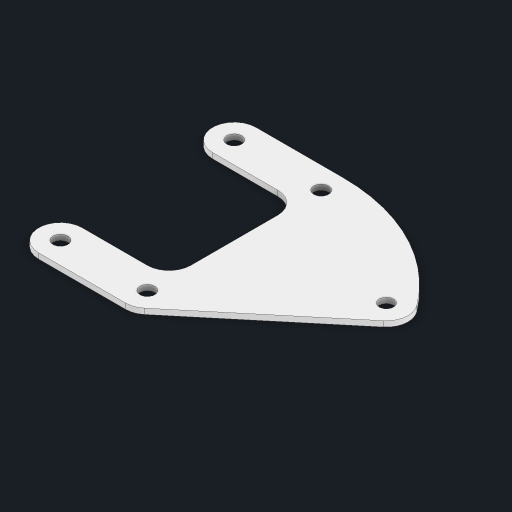
# Autodesk Inventor part: gusset
Saved by Autodesk Inventor 2024 (Build 280153000, 153)
## iProperties
Created: 2024-03-02
Part Number: gusset
Material: Acetal Resin, White
Document SubType Name: Modeling
Designer: Averey Ku
Density: 1.425 g/cm^3
Appearance: Smooth - White
d0: 0.250 in
Author: Averey Ku
Autodesk Inventor part; units mm, degrees
ref_plane "YZ Plane" through (0, 0, 0) normal (1, 0, 0) x (0, 1, 0)
ref_plane "XZ Plane" through (0, 0, 0) normal (0, 1, 0) x (-1, 0, 0)
ref_plane "XY Plane" through (0, 0, 0) normal (0, 0, 1) x (1, 0, 0)
sketch "main" plane through (0, 0, 0) normal (0, 0, 1) x (1, 0, 0)
  circle A0 centre (33.5416, 32.0006) radius 2.1844
  line L0 (8.1416, 38.3506) -> (33.5416, 38.3506)
  line L1 (33.5416, 25.6506) -> (14.4916, 25.6506)
  arc A1 (33.5416, 25.6506) -> (33.5416, 38.3506) centre (33.5416, 32.0006) ccw
  circle A2 centre (8.1416, 32.0006) radius 2.1844
  arc A3 (14.4916, 25.6506) -> (8.1416, 19.3006) centre (14.4916, 19.3006) ccw
  arc A4 (8.1416, 38.3506) -> (4.0764, 36.8788) centre (8.1416, 32.0006) ccw
  circle A5 centre (33.5416, -18.7994) radius 2.1844
  line L2 (8.1416, -6.0994) -> (8.1416, 19.3006)
  arc A6 (8.1416, -6.0994) -> (14.4916, -12.4494) centre (14.4916, -6.0994) ccw
  circle A7 centre (8.1416, -18.7994) radius 2.1844
  line L3 (-34.0236, 5.1288) -> (4.0764, 36.8788)
  circle A8 centre (-29.9584, 0.2506) radius 2.0955
  arc A9 (-35.0384, -3.5594) -> (8.1416, -25.1494) centre (8.1416, 28.8256) ccw
  arc A10 (-34.0236, 5.1288) -> (-35.0384, -3.5594) centre (-29.9584, 0.2506) ccw
  line L4 (14.4916, -12.4494) -> (33.5416, -12.4494)
  line L5 (8.1416, -25.1494) -> (33.5416, -25.1494)
  arc A11 (33.5416, -25.1494) -> (33.5416, -12.4494) centre (33.5416, -18.7994) ccw
  point P0 (9.5067, 8.1196)
  point P1 (8.1416, 25.6506)
  point P2 (8.1416, -12.4494)
  dimension "d0" = 6.35
  measures "d0" radius of A3
sketch "Sketch1" plane through (0, 0, 0) normal (0, 1, 0) x (-1, 0, 0)
  circle A0 centre (0, 0) radius 2.1844
  line L0 (-25.4, 6.35) -> (0, 6.35)
  line L1 (0, -6.35) -> (-19.05, -6.35)
  arc A1 (0, -6.35) -> (0, 6.35) centre (0, 0) ccw
  circle A2 centre (-25.4, 0) radius 2.1844
  arc A3 (-19.05, -6.35) -> (-25.4, -12.7) centre (-19.05, -12.7) ccw
  arc A4 (-25.4, 6.35) -> (-29.4652, 4.8782) centre (-25.4, 0) ccw
  circle A5 centre (0, -50.8) radius 2.1844
  line L2 (-25.4, -38.1) -> (-25.4, -12.7)
  arc A6 (-25.4, -38.1) -> (-19.05, -44.45) centre (-19.05, -38.1) ccw
  circle A7 centre (-25.4, -50.8) radius 2.1844
  line L3 (-67.5652, -26.8718) -> (-29.4652, 4.8782)
  circle A8 centre (-63.5, -31.75) radius 2.0955
  arc A9 (-68.58, -35.56) -> (-25.4, -57.15) centre (-25.4, -3.175) ccw
  arc A10 (-67.5652, -26.8718) -> (-68.58, -35.56) centre (-63.5, -31.75) ccw
  line L4 (-19.05, -44.45) -> (0, -44.45)
  line L5 (-25.4, -57.15) -> (0, -57.15)
  arc A11 (0, -57.15) -> (0, -44.45) centre (0, -50.8) ccw
  constraints: 1 other
extrude "Extrusion1" add sketch "Sketch1" along normal blind 1.5875
body "Solid1"
